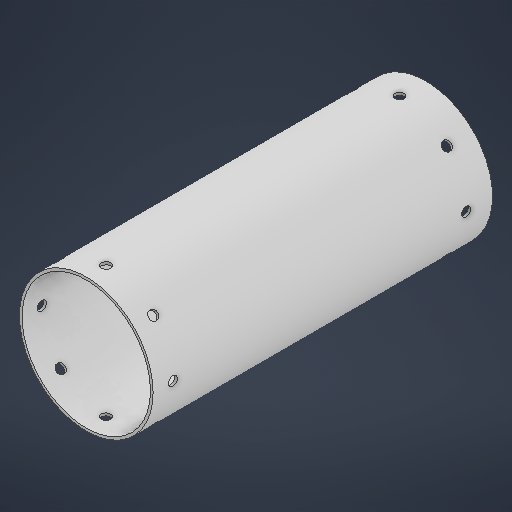
# Autodesk Inventor part: casing 258mm
Saved by Autodesk Inventor 2027 (Build 310192060, 192F)
## iProperties
Created: 2026-06-29
Part Number: casing 258mm
Material: Generic
Document SubType Name: Modeling
Designer: Alex T. Wandugu
Density: 1 g/cm^3
Appearance: Default
Matter: Aluminium
Author: Alex T. Wandugu
Autodesk Inventor part; units mm, degrees
ref_plane "YZ Plane" through (0, 0, 0) normal (1, 0, 0) x (0, 1, 0)
ref_plane "XZ Plane" through (0, 0, 0) normal (0, 1, 0) x (-1, 0, 0)
ref_plane "XY Plane" through (0, 0, 0) normal (0, 0, 1) x (1, 0, 0)
sketch "Sketch1" plane through (0, 0, 0) normal (0, 0, 1) x (1, 0, 0)
  circle A0 centre (0, 0) radius 50.8
  circle A1 centre (0, 0) radius 48.8
  dimension "d0" = 101.6
  dimension "d1" = 97.6
  constraints: 2 centre point, 2 coincident
  measures "d0" diameter of A0
  measures "d1" diameter of A1
extrude "Extrusion1" add sketch "Sketch1" against normal blind 258
sketch "Sketch3" plane through (0, 0, 0) normal (1, 0, 0) x (0, 1, 0)
  line L0 (-48.8, 0) -> (48.8, 0) projected
  line L1 (0, 0) -> (0, -15)
  line L2 (48.8, -258) -> (-48.8, -258) projected
  line L3 (0, -258) -> (0, -238)
  circle A0 centre (0, -15) radius 3.5
  circle A1 centre (0, -238) radius 3.5
  dimension "d10" = 15
  dimension "d11" = 20
  dimension "d12" = 7
  dimension "d13" = 7
  constraints: 4 end point, 2 centre point, 2 coincident, 2 vertical, 1 midpoint
  measures "d10" distance of L1.start L1.end
  measures "d11" distance of L3.start L3.end
  measures "d12" diameter of A0
  measures "d13" diameter of A1
extrude "Extrusion3" cut sketch "Sketch3" along normal through all both and the other way through all
pattern_circular "Circular Pattern2" count 8 over 360 about axis through (0, 0, -10) along (0, 0, 1) of "Extrusion3"
body "Solid1"
